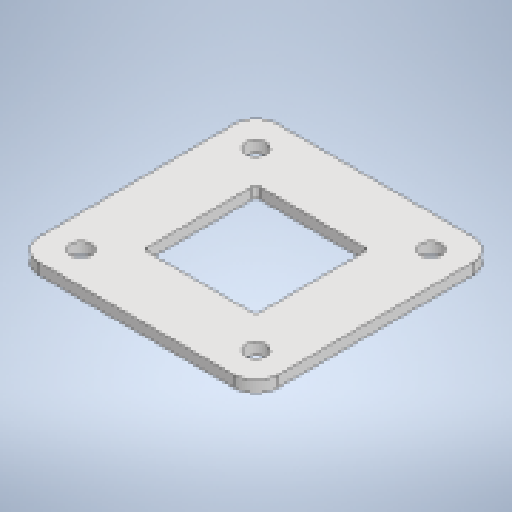
# Autodesk Inventor part: ANP 1425 FDS Way FLANGE
Saved by Autodesk Inventor 2025 (Build 290162010, 162A)
## iProperties
Created: 2025-06-24
Part Number: ANP 1425 FDS Way FLANGE
Material: Stainless Steel
Document SubType Name: Sheet Metal
Designer: user
Mass: 103.446 g
Surface Area: 101.897 cm^2
Volume: 12.9307 cm^3
Density: 8 g/cm^3
Sheet Metal Rule: AISI304 2mm Die16
Sheet Metal Width: 64,200 mm
Sheet Metal Length: 64,200 mm
Sheet Metal Area: 4121,640 mm^2
Appearance: Default
Flat Pattern Width: 6.42 cm
Flat Pattern Length: 6.42 cm
Flat Pattern Area: 41.2164 cm^2
Author: user
Autodesk Inventor part; units mm, degrees
ref_plane "YZ Plane" through (0, 0, 0) normal (1, 0, 0) x (0, 1, 0)
ref_plane "XZ Plane" through (0, 0, 0) normal (0, 1, 0) x (-1, 0, 0)
ref_plane "XY Plane" through (0, 0, 0) normal (0, 0, 1) x (1, 0, 0)
sketch "Sketch1" plane through (0, 0, 0) normal (0, 0, 1) x (1, 0, 0)
  line L0 (-32.1, -32.1) -> (32.1, -32.1)
  line L1 (32.1, -32.1) -> (32.1, 32.1)
  line L2 (32.1, 32.1) -> (-32.1, 32.1)
  line L3 (-32.1, 32.1) -> (-32.1, -32.1)
  line L4 (-32.1, -32.1) -> (32.1, 32.1) construction
  line L5 (32.1, -32.1) -> (-32.1, 32.1) construction
  line L6 (15.1, -15.1) -> (-15.1, -15.1)
  line L7 (-15.1, -15.1) -> (-15.1, 15.1)
  line L8 (-15.1, 15.1) -> (15.1, 15.1)
  line L9 (15.1, 15.1) -> (15.1, -15.1)
  line L10 (15.1, -15.1) -> (-15.1, 15.1) construction
  line L11 (-15.1, -15.1) -> (15.1, 15.1) construction
  point P0 (0, 0)
  dimension "d172" = 30.2
  dimension "d181" = 17
  dimension "d187" = 17
  measures "d172" distance of L7.end L8.end
  measures "d181" distance between parallel lines of L1 L9
  measures "d187" distance between parallel lines of L2 L8
extrude "Plate5" add sketch "Sketch1" along normal blind 3
sketch "Sketch9" plane through (0, 0, 3) normal (0, 0, 1) x (1, 0, 0)
  circle A0 centre (23.4853, -23.4853) radius 2.75
  line L0 (23.4853, 23.4853) -> (-23.4853, 23.4853) construction
  line L1 (-23.4853, 23.4853) -> (-23.4853, -23.4853) construction
  line L2 (-23.4853, -23.4853) -> (23.4853, -23.4853) construction
  line L3 (23.4853, -23.4853) -> (23.4853, 23.4853) construction
  line L4 (23.4853, 23.4853) -> (-23.4853, -23.4853) construction
  line L5 (-23.4853, 23.4853) -> (23.4853, -23.4853) construction
  circle A1 centre (-23.4853, -23.4853) radius 2.75
  circle A2 centre (23.4853, 23.4853) radius 2.75
  circle A3 centre (-23.4853, 23.4853) radius 2.75
  circle A4 centre (0, 0) radius 33.2132 construction
  line L6 (-15.1, -15.1) -> (-15.1, 15.1) projected
  line L7 (-15.1, 15.1) -> (15.1, 15.1) projected
  line L8 (15.1, 15.1) -> (15.1, -15.1) projected
  line L9 (15.1, -15.1) -> (-15.1, -15.1) projected
  line L10 (32.1, -32.1) -> (-32.1, -32.1) projected
  line L11 (32.1, 32.1) -> (32.1, -32.1) projected
  line L12 (-32.1, 32.1) -> (32.1, 32.1) projected
  line L13 (-32.1, -32.1) -> (-32.1, 32.1) projected
  line L14 (-15, 15) -> (15, 15) construction
  line L15 (15, 15) -> (15, -15) construction
  line L16 (15, -15) -> (-15, -15) construction
  line L17 (-15, -15) -> (-15, 15) construction
  line L18 (-15, -15) -> (15, 15) construction
  dimension "d174" = 5.5
  dimension "d184" = 30
  dimension "d185" = 30
  dimension "d186" = 12
  constraints: 22 end point, 8 coincident, 4 centre point, 4 parallel, 3 equal radius, 3 midpoint, 3 perpendicular, 2 horizontal, 3 other
  measures "d174" diameter of A0
  measures "d184" distance of L14.start L14.end
  measures "d185" distance of L14.end L15.end
  measures "d186" distance of L0.end L14.start
extrude "Cut2" cut sketch "Sketch9" against normal blind 3 contours A0 | A1 | A2 | A3
fillet "Corner Round1" radius 6 4 edges at (32.1, 32.1, 1.5) (-32.1, 32.1, 1.5) (-32.1, -32.1, 1.5) (32.1, -32.1, 1.5)
fillet "Corner Round2" radius 1 4 edges at (-15.1, 15.1, 1.5) (-15.1, -15.1, 1.5) (15.1, -15.1, 1.5) (15.1, 15.1, 1.5)
body "Solid3"
